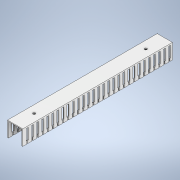
# Autodesk Inventor part: Cablecanal Ranurado 30x30 L=100 mm
Saved by Autodesk Inventor 2020 (Build 240168000, 168)
## iProperties
Created: 2020-07-11
Part Number: Cablecanal Ranurado 30x30 L=100 mm
Material: PPS Plastic
Document SubType Name: Modeling
Designer: Hernan
Density: 1.637 g/cm^3
Appearance: Smooth - White
Author: Hernan
Autodesk Inventor part; units mm, degrees
ref_plane "YZ Plane" through (0, 0, 0) normal (1, 0, 0) x (0, 1, 0)
ref_plane "XZ Plane" through (0, 0, 0) normal (0, 1, 0) x (-1, 0, 0)
ref_plane "XY Plane" through (0, 0, 0) normal (0, 0, 1) x (1, 0, 0)
sketch "Sketch1" plane through (0, 0, 0) normal (0, 0, 1) x (1, 0, 0)
  line L0 (-11.9963, 7.4108) -> (18.0037, 7.4108)
  line L1 (18.0037, 7.4108) -> (18.0037, -22.5892)
  line L2 (18.0037, -22.5892) -> (-11.9963, -22.5892)
  line L3 (-11.9963, -22.5892) -> (-11.9963, 7.4108)
  line L4 (16.3037, 5.7108) -> (-10.2963, 5.7108)
  line L5 (-10.2963, 5.7108) -> (-10.2963, -22.5892)
  line L6 (-10.2963, -20.8892) -> (16.3037, -20.8892)
  line L7 (16.3037, -22.5892) -> (16.3037, 5.7108)
  point P0 (0, 0)
  dimension "d0" = 30
  dimension "d1" = 30
  dimension "d2" = 1.7
  constraints: 16 end point, 4 parallel, 4 point on line, 2 perpendicular, 1 horizontal
  measures "d0" distance of L0.start L0.end
  measures "d1" distance of L0.end L1.end
  measures "d2" distance between parallel lines of L0 L4
extrude "Extrusion1" add sketch "Sketch1" against normal blind 294.879
extrude "Extrusion2" cut sketch "Sketch1" against normal blind 300 contours L5 L6 L7 L2 | L5 L4 L7 L6
sketch "Boceto2" plane through (-11.9963, 7.4108, 0) normal (0, 1, 0) x (1, 0, 0)
  line L0 (0, 294.879) -> (30, 294.879) projected
  line L1 (28.3, 0) -> (1.7, 0) projected
  circle A0 centre (15, 37.3509) radius 2.5
  circle A1 centre (15, 257.3509) radius 2.5
  point P0 (11.9963, 0)
  dimension "d7" = 5
  dimension "d8" = 5
  dimension "d12" = 220
  constraints: 2 centre point
  measures "d7" diameter of A0
  measures "d8" diameter of A1
  measures "d12" distance of A0.centre A1.centre
extrude "Extrusión3" cut sketch "Boceto2" against normal blind 10
sketch "Boceto3" plane through (-11.9963, -22.5892, 0) normal (-1, 0, 0) x (0, 0, 1)
  line L0 (0, 30) -> (0, 0) projected
  line L1 (0, 0) -> (-8, 0)
  line L2 (0, 0) -> (-294.879, 0) projected
  line L3 (-8, 0) -> (-8, 5)
  line L4 (-7, 6.5) -> (-7, 27.1667)
  line L5 (0, 30) -> (-294.879, 30) projected
  line L6 (0, 0) -> (0, 5)
  line L7 (-1, 6.5) -> (-1, 27.1667)
  line L8 (0, 5) -> (-1, 6.5)
  line L9 (-7, 6.5) -> (-8, 5)
  line L10 (-10, 0) -> (-18, 0)
  line L11 (-18, 0) -> (-18, 5)
  line L12 (-17, 6.5) -> (-17, 27.1667)
  line L13 (-10, 0) -> (-10, 5)
  line L14 (-11, 6.5) -> (-11, 27.1667)
  line L15 (-10, 5) -> (-11, 6.5)
  line L16 (-17, 6.5) -> (-18, 5)
  line L17 (-20, 0) -> (-28, 0)
  line L18 (-28, 0) -> (-28, 5)
  line L19 (-27, 6.5) -> (-27, 27.1667)
  line L20 (-20, 0) -> (-20, 5)
  line L21 (-21, 6.5) -> (-21, 27.1667)
  line L22 (-20, 5) -> (-21, 6.5)
  line L23 (-27, 6.5) -> (-28, 5)
  line L24 (-30, 0) -> (-38, 0)
  line L25 (-38, 0) -> (-38, 5)
  line L26 (-37, 6.5) -> (-37, 27.1667)
  line L27 (-30, 0) -> (-30, 5)
  line L28 (-31, 6.5) -> (-31, 27.1667)
  line L29 (-30, 5) -> (-31, 6.5)
  line L30 (-37, 6.5) -> (-38, 5)
  line L31 (-40, 0) -> (-48, 0)
  line L32 (-48, 0) -> (-48, 5)
  line L33 (-47, 6.5) -> (-47, 27.1667)
  line L34 (-40, 0) -> (-40, 5)
  line L35 (-41, 6.5) -> (-41, 27.1667)
  line L36 (-40, 5) -> (-41, 6.5)
  line L37 (-47, 6.5) -> (-48, 5)
  line L38 (-50, 0) -> (-58, 0)
  line L39 (-58, 0) -> (-58, 5)
  line L40 (-57, 6.5) -> (-57, 27.1667)
  line L41 (-50, 0) -> (-50, 5)
  line L42 (-51, 6.5) -> (-51, 27.1667)
  line L43 (-50, 5) -> (-51, 6.5)
  line L44 (-57, 6.5) -> (-58, 5)
  line L45 (-60, 0) -> (-68, 0)
  line L46 (-68, 0) -> (-68, 5)
  line L47 (-67, 6.5) -> (-67, 27.1667)
  line L48 (-60, 0) -> (-60, 5)
  line L49 (-61, 6.5) -> (-61, 27.1667)
  line L50 (-60, 5) -> (-61, 6.5)
  line L51 (-67, 6.5) -> (-68, 5)
  line L52 (-70, 0) -> (-78, 0)
  line L53 (-78, 0) -> (-78, 5)
  line L54 (-77, 6.5) -> (-77, 27.1667)
  line L55 (-70, 0) -> (-70, 5)
  line L56 (-71, 6.5) -> (-71, 27.1667)
  line L57 (-70, 5) -> (-71, 6.5)
  line L58 (-77, 6.5) -> (-78, 5)
  line L59 (-80, 0) -> (-88, 0)
  line L60 (-88, 0) -> (-88, 5)
  line L61 (-87, 6.5) -> (-87, 27.1667)
  line L62 (-80, 0) -> (-80, 5)
  line L63 (-81, 6.5) -> (-81, 27.1667)
  line L64 (-80, 5) -> (-81, 6.5)
  line L65 (-87, 6.5) -> (-88, 5)
  line L66 (-90, 0) -> (-98, 0)
  line L67 (-98, 0) -> (-98, 5)
  line L68 (-97, 6.5) -> (-97, 27.1667)
  line L69 (-90, 0) -> (-90, 5)
  line L70 (-91, 6.5) -> (-91, 27.1667)
  line L71 (-90, 5) -> (-91, 6.5)
  line L72 (-97, 6.5) -> (-98, 5)
  line L73 (-100, 0) -> (-108, 0)
  line L74 (-108, 0) -> (-108, 5)
  line L75 (-107, 6.5) -> (-107, 27.1667)
  line L76 (-100, 0) -> (-100, 5)
  line L77 (-101, 6.5) -> (-101, 27.1667)
  line L78 (-100, 5) -> (-101, 6.5)
  line L79 (-107, 6.5) -> (-108, 5)
  line L80 (-110, 0) -> (-118, 0)
  line L81 (-118, 0) -> (-118, 5)
  line L82 (-117, 6.5) -> (-117, 27.1667)
  line L83 (-110, 0) -> (-110, 5)
  line L84 (-111, 6.5) -> (-111, 27.1667)
  line L85 (-110, 5) -> (-111, 6.5)
  line L86 (-117, 6.5) -> (-118, 5)
  line L87 (-120, 0) -> (-128, 0)
  line L88 (-128, 0) -> (-128, 5)
  line L89 (-127, 6.5) -> (-127, 27.1667)
  line L90 (-120, 0) -> (-120, 5)
  line L91 (-121, 6.5) -> (-121, 27.1667)
  line L92 (-120, 5) -> (-121, 6.5)
  line L93 (-127, 6.5) -> (-128, 5)
  line L94 (-130, 0) -> (-138, 0)
  line L95 (-138, 0) -> (-138, 5)
  line L96 (-137, 6.5) -> (-137, 27.1667)
  line L97 (-130, 0) -> (-130, 5)
  line L98 (-131, 6.5) -> (-131, 27.1667)
  line L99 (-130, 5) -> (-131, 6.5)
  line L100 (-137, 6.5) -> (-138, 5)
  line L101 (-140, 0) -> (-148, 0)
  line L102 (-148, 0) -> (-148, 5)
  line L103 (-147, 6.5) -> (-147, 27.1667)
  line L104 (-140, 0) -> (-140, 5)
  line L105 (-141, 6.5) -> (-141, 27.1667)
  line L106 (-140, 5) -> (-141, 6.5)
  line L107 (-147, 6.5) -> (-148, 5)
  line L108 (-150, 0) -> (-158, 0)
  line L109 (-158, 0) -> (-158, 5)
  line L110 (-157, 6.5) -> (-157, 27.1667)
  line L111 (-150, 0) -> (-150, 5)
  line L112 (-151, 6.5) -> (-151, 27.1667)
  line L113 (-150, 5) -> (-151, 6.5)
  line L114 (-157, 6.5) -> (-158, 5)
  line L115 (-160, 0) -> (-168, 0)
  line L116 (-168, 0) -> (-168, 5)
  line L117 (-167, 6.5) -> (-167, 27.1667)
  line L118 (-160, 0) -> (-160, 5)
  line L119 (-161, 6.5) -> (-161, 27.1667)
  line L120 (-160, 5) -> (-161, 6.5)
  line L121 (-167, 6.5) -> (-168, 5)
  line L122 (-170, 0) -> (-178, 0)
  line L123 (-178, 0) -> (-178, 5)
  line L124 (-177, 6.5) -> (-177, 27.1667)
  line L125 (-170, 0) -> (-170, 5)
  line L126 (-171, 6.5) -> (-171, 27.1667)
  line L127 (-170, 5) -> (-171, 6.5)
  line L128 (-177, 6.5) -> (-178, 5)
  line L129 (-180, 0) -> (-188, 0)
  line L130 (-188, 0) -> (-188, 5)
  line L131 (-187, 6.5) -> (-187, 27.1667)
  line L132 (-180, 0) -> (-180, 5)
  line L133 (-181, 6.5) -> (-181, 27.1667)
  line L134 (-180, 5) -> (-181, 6.5)
  line L135 (-187, 6.5) -> (-188, 5)
  line L136 (-190, 0) -> (-198, 0)
  line L137 (-198, 0) -> (-198, 5)
  line L138 (-197, 6.5) -> (-197, 27.1667)
  line L139 (-190, 0) -> (-190, 5)
  line L140 (-191, 6.5) -> (-191, 27.1667)
  line L141 (-190, 5) -> (-191, 6.5)
  line L142 (-197, 6.5) -> (-198, 5)
  line L143 (-200, 0) -> (-208, 0)
  line L144 (-208, 0) -> (-208, 5)
  line L145 (-207, 6.5) -> (-207, 27.1667)
  line L146 (-200, 0) -> (-200, 5)
  line L147 (-201, 6.5) -> (-201, 27.1667)
  line L148 (-200, 5) -> (-201, 6.5)
  line L149 (-207, 6.5) -> (-208, 5)
  line L150 (-210, 0) -> (-218, 0)
  line L151 (-218, 0) -> (-218, 5)
  line L152 (-217, 6.5) -> (-217, 27.1667)
  line L153 (-210, 0) -> (-210, 5)
  line L154 (-211, 6.5) -> (-211, 27.1667)
  line L155 (-210, 5) -> (-211, 6.5)
  line L156 (-217, 6.5) -> (-218, 5)
  line L157 (-220, 0) -> (-228, 0)
  line L158 (-228, 0) -> (-228, 5)
  line L159 (-227, 6.5) -> (-227, 27.1667)
  line L160 (-220, 0) -> (-220, 5)
  line L161 (-221, 6.5) -> (-221, 27.1667)
  line L162 (-220, 5) -> (-221, 6.5)
  line L163 (-227, 6.5) -> (-228, 5)
  line L164 (-230, 0) -> (-238, 0)
  line L165 (-238, 0) -> (-238, 5)
  line L166 (-237, 6.5) -> (-237, 27.1667)
  line L167 (-230, 0) -> (-230, 5)
  line L168 (-231, 6.5) -> (-231, 27.1667)
  line L169 (-230, 5) -> (-231, 6.5)
  line L170 (-237, 6.5) -> (-238, 5)
  line L171 (-240, 0) -> (-248, 0)
  line L172 (-248, 0) -> (-248, 5)
  line L173 (-247, 6.5) -> (-247, 27.1667)
  line L174 (-240, 0) -> (-240, 5)
  line L175 (-241, 6.5) -> (-241, 27.1667)
  line L176 (-240, 5) -> (-241, 6.5)
  line L177 (-247, 6.5) -> (-248, 5)
  line L178 (-250, 0) -> (-258, 0)
  line L179 (-258, 0) -> (-258, 5)
  line L180 (-257, 6.5) -> (-257, 27.1667)
  line L181 (-250, 0) -> (-250, 5)
  line L182 (-251, 6.5) -> (-251, 27.1667)
  line L183 (-250, 5) -> (-251, 6.5)
  line L184 (-257, 6.5) -> (-258, 5)
  line L185 (-260, 0) -> (-268, 0)
  line L186 (-268, 0) -> (-268, 5)
  line L187 (-267, 6.5) -> (-267, 27.1667)
  line L188 (-260, 0) -> (-260, 5)
  line L189 (-261, 6.5) -> (-261, 27.1667)
  line L190 (-260, 5) -> (-261, 6.5)
  line L191 (-267, 6.5) -> (-268, 5)
  line L192 (-277, 6.5) -> (-277, 27.1667)
  line L193 (-271, 6.5) -> (-271, 27.1667)
  line L194 (-270, 5) -> (-271, 6.5)
  line L195 (-270, 0) -> (-270, 5)
  line L196 (-278, 0) -> (-278, 5)
  line L197 (-277, 6.5) -> (-278, 5)
  line L198 (-270, 0) -> (-278, 0)
  line L199 (-287, 6.5) -> (-287, 27.1667)
  line L200 (-281, 6.5) -> (-281, 27.1667)
  line L201 (-280, 5) -> (-281, 6.5)
  line L202 (-280, 0) -> (-280, 5)
  line L203 (-288, 0) -> (-288, 5)
  line L204 (-287, 6.5) -> (-288, 5)
  line L205 (-280, 0) -> (-288, 0)
  line L206 (-291, 6.5) -> (-291, 27.1667)
  line L207 (-290, 5) -> (-291, 6.5)
  line L208 (-290, 0) -> (-290, 5)
  line L209 (-290, 0) -> (-294.879, 0)
  line L210 (0, 27.1667) -> (-291, 27.1667)
  point P0 (0, 22.5892)
  point P1 (-290, 0)
  dimension "d15" = 8
  dimension "d20" = 8
  dimension "d21" = 8
  dimension "d22" = 8
  dimension "d23" = 8
  dimension "d24" = 8
  dimension "d25" = 8
  dimension "d26" = 8
  dimension "d27" = 8
  dimension "d28" = 8
  dimension "d29" = 8
  dimension "d30" = 8
  dimension "d31" = 8
  dimension "d32" = 8
  dimension "d33" = 8
  dimension "d34" = 8
  dimension "d35" = 8
  dimension "d36" = 8
  dimension "d37" = 8
  dimension "d38" = 8
  dimension "d39" = 8
  dimension "d40" = 8
  dimension "d41" = 8
  dimension "d42" = 8
  dimension "d43" = 8
  dimension "d44" = 8
  dimension "d45" = 8
  dimension "d46" = 2
  dimension "d47" = 2
  dimension "d48" = 2
  dimension "d49" = 2
  dimension "d50" = 2
  dimension "d51" = 2
  dimension "d52" = 2
  dimension "d53" = 2
  dimension "d54" = 2
  dimension "d55" = 2
  dimension "d56" = 2
  dimension "d57" = 2
  dimension "d58" = 2
  dimension "d59" = 2
  dimension "d60" = 2
  dimension "d61" = 2
  dimension "d62" = 2
  dimension "d63" = 2
  dimension "d64" = 2
  dimension "d65" = 2
  dimension "d66" = 2
  dimension "d67" = 2
  dimension "d68" = 2
  dimension "d69" = 2
  dimension "d70" = 2
  dimension "d71" = 2
  dimension "d72" = 8
  dimension "d73" = 8
  dimension "d75" = 2
  dimension "d76" = 2
  dimension "d78" = 2
  constraints: 414 end point, 29 parallel, 29 perpendicular, 1 horizontal, 1 point on line, 63 other
  measures "d15" distance of L0.end L1.end
  measures "d20" distance of L13.start L11.start
  measures "d21" distance of L20.start L18.start
  measures "d22" distance of L27.start L25.start
  measures "d23" distance of L34.start L32.start
  measures "d24" distance of L41.start L39.start
  measures "d25" distance of L48.start L46.start
  measures "d26" distance of L55.start L53.start
  measures "d27" distance of L62.start L60.start
  measures "d28" distance of L69.start L67.start
  measures "d29" distance of L76.start L74.start
  measures "d30" distance of L83.start L81.start
  measures "d31" distance of L90.start L88.start
  measures "d32" distance of L97.start L95.start
  measures "d33" distance of L104.start L102.start
  measures "d34" distance of L111.start L109.start
  measures "d35" distance of L118.start L116.start
  measures "d36" distance of L125.start L123.start
  measures "d37" distance of L132.start L130.start
  measures "d38" distance of L139.start L137.start
  measures "d39" distance of L146.start L144.start
  measures "d40" distance of L153.start L151.start
  measures "d41" distance of L160.start L158.start
  measures "d42" distance of L167.start L165.start
  measures "d43" distance of L174.start L172.start
  measures "d44" distance of L181.start L179.start
  measures "d45" distance of L188.start L186.start
  measures "d46" distance of L13.start L1.end
  measures "d47" distance of L20.start L11.start
  measures "d48" distance of L27.start L18.start
  measures "d49" distance of L34.start L25.start
  measures "d50" distance of L41.start L32.start
  measures "d51" distance of L48.start L39.start
  measures "d52" distance of L55.start L46.start
  measures "d53" distance of L62.start L53.start
  measures "d54" distance of L69.start L60.start
  measures "d55" distance of L76.start L67.start
  measures "d56" distance of L83.start L74.start
  measures "d57" distance of L90.start L81.start
  measures "d58" distance of L97.start L88.start
  measures "d59" distance of L104.start L95.start
  measures "d60" distance of L111.start L102.start
  measures "d61" distance of L118.start L109.start
  measures "d62" distance of L125.start L116.start
  measures "d63" distance of L132.start L123.start
  measures "d64" distance of L139.start L130.start
  measures "d65" distance of L146.start L137.start
  measures "d66" distance of L153.start L144.start
  measures "d67" distance of L160.start L151.start
  measures "d68" distance of L167.start L158.start
  measures "d69" distance of L174.start L165.start
  measures "d70" distance of L181.start L172.start
  measures "d71" distance of L188.start L179.start
  measures "d72" distance of L195.start L196.start
  measures "d73" distance of L202.start L203.start
  measures "d75" distance of L195.start L186.start
  measures "d76" distance of L202.start L196.start
  measures "d78" distance between parallel lines of L203 L208
extrude "Extrusión4" cut sketch "Boceto3" against normal blind 30 contours L4 L9 L3 L2 L13 L15 L14 L210 | L12 L16 L11 L2 L20 L22 L21 L210 | L19 L23 L18 L2 L27 L29 L28 L210 | L26 L30 L25 L2 L34 L36 L35 L210 | L33 L37 L32 L2 L41 L43 L42 L210 | L40 L44 L39 L2 L48 L50 L49 L210 | L47 L51 L46 L2 L55 L57 L56 L210 | L54 L58 L53 L2 L62 L64 L63 L210 | L61 L65 L60 L2 L69 L71 L70 L210 | L68 L72 L67 L2 L76 L78 L77 L210 | L75 L79 L74 L2 L83 L85 L84 L210 | L82 L86 L81 L2 L90 L92 L91 L210 | L89 L93 L88 L2 L97 L99 L98 L210 | L96 L100 L95 L2 L104 L106 L105 L210 | L103 L107 L102 L2 L111 L113 L112 L210 | L110 L114 L109 L2 L118 L120 L119 L210 | L117 L121 L116 L2 L125 L127 L126 L210 | L124 L128 L123 L2 L132 L134 L133 L210 | L131 L135 L130 L2 L139 L141 L140 L210 | L138 L142 L137 L2 L146 L148 L147 L210 | L145 L149 L144 L2 L153 L155 L154 L210 | L152 L156 L151 L2 L160 L162 L161 L210 | L159 L163 L158 L2 L167 L169 L168 L210 | L166 L170 L165 L2 L174 L176 L175 L210 | L173 L177 L172 L2 L181 L183 L182 L210 | L180 L184 L179 L2 L188 L190 L189 L210 | L187 L191 L186 L2 L195 L194 L193 L210 | L192 L197 L196 L2 L202 L201 L200 L210 | L199 L204 L203 L2 L208 L207 L206 L210
body "Solid1"
